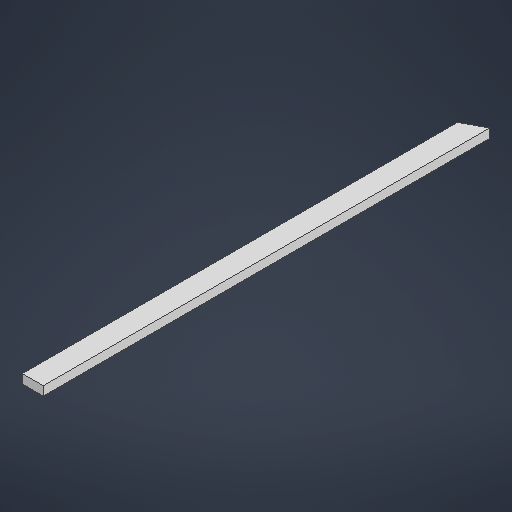
# Autodesk Inventor part: S_2x4x96
Saved by Autodesk Inventor 2027.1 (Build 311270010, 270A)
## iProperties
Created: 2026-09-01
Part Number: S_2x4x96
Material: Generic
Document SubType Name: Modeling
Designer: jorda
Density: 1 g/cm^3
Appearance: Default
Author: jorda
Autodesk Inventor part; units mm, degrees
ref_plane "YZ Plane" through (0, 0, 0) normal (1, 0, 0) x (0, 1, 0)
ref_plane "XZ Plane" through (0, 0, 0) normal (0, 1, 0) x (-1, 0, 0)
ref_plane "XY Plane" through (0, 0, 0) normal (0, 0, 1) x (1, 0, 0)
sketch "Sketch1" plane through (0, 0, 0) normal (0, 1, 0) x (-1, 0, 0)
  line L0 (88.9, -545.084) -> (88.9, -2391.131)
  line L1 (0, -2438.4) -> (88.9, -2391.131)
  line L2 (0, -2438.4) -> (107.992, -2438.4) construction
  line L3 (0, -2438.4) -> (0, -545.084)
  line L4 (0, -2438.4) -> (0, -545.084)
  line L5 (0, -2438.4) -> (0, -545.084)
  line L6 (0, -545.084) -> (88.9, -545.084)
  point P0 (0, 0)
  constraints: 14 end point, 1 horizontal, 1 perpendicular
extrude "Extrusion1" add sketch "Sketch1" along normal blind 38.1
body "Solid1"
